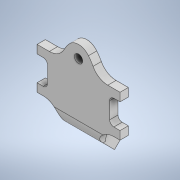
# Autodesk Inventor part: led_cap
Saved by Autodesk Inventor 2022 (Build 260153000, 153)
## iProperties
Created: 2024-07-06
Part Number: led_cap
Material: Типовые
Document SubType Name: Modeling
Designer: Капустяник Андрей
Density: 1 g/cm^3
Appearance: По умолчанию
Author: Капустяник Андрей
Autodesk Inventor part; units mm, degrees
ref_plane "YZ Plane" through (0, 0, 0) normal (1, 0, 0) x (0, 1, 0)
ref_plane "XZ Plane" through (0, 0, 0) normal (0, 1, 0) x (-1, 0, 0)
ref_plane "XY Plane" through (0, 0, 0) normal (0, 0, 1) x (1, 0, 0)
sketch "Эскиз1" plane through (0, 0, 0) normal (0, 0, 1) x (1, 0, 0)
  circle A0 centre (0, 0) radius 4.25
  line L0 (-4.5, 10) -> (4.5, 10)
  line L1 (4.5, 10) -> (4.5, -10)
  line L2 (4.5, -10) -> (-4.5, -10)
  line L3 (-4.5, -10) -> (-4.5, 10)
  line L4 (-4.5, 10) -> (4.5, -10) construction
  line L5 (4.5, 10) -> (-4.5, -10) construction
  dimension "d0" = 8.5
  dimension "d1" = 9
  dimension "d2" = 20
  constraints: 12 end point, 2 midpoint, 2 parallel, 1 centre point, 1 coincident, 1 horizontal, 1 perpendicular
  measures "d0" diameter of A0
  measures "d1" distance of L1.end L2.end
  measures "d2" distance of L0.end L1.end
extrude "Выдавливание1" add sketch "Эскиз1" along normal blind 2 contours A0 | L0 L1 L2 L3
sketch "Эскиз2" plane through (4.5, -10, 0) normal (1, 0, 0) x (0, 0, -1)
  line L0 (1.1161, 0) -> (2.1768, -1.0607) projected
  line L1 (3.9445, 0.7071) -> (2.1768, -1.0607) projected
  line L2 (3.9445, 0.7071) -> (2, 2.6517) projected
  line L3 (1.3283, 0.2121) -> (2.1768, -0.6364)
  line L4 (2.1768, -0.6364) -> (3.5203, 0.7071)
  line L5 (3.5203, 0.7071) -> (1.7879, 2.4395)
  line L6 (1.3283, 0.2121) -> (0, 1.5404)
  line L7 (0, 0) -> (0, 20) projected
  line L8 (1.7879, 2.4395) -> (0, 4.2274)
  point P0 (0, 10)
  dimension "d5" = 0.3
  constraints: 10 end point, 2 collinear, 2 point on line, 2 other
  measures "d5" distance between parallel lines of L1 L4
extrude "Выдавливание2" add sketch "Эскиз2" against normal up to surface (9 mm away)
sketch "Эскиз3" plane through (-4.5, -10, 2) normal (-1, 0, 0) x (0, 0, 1)
  line L0 (-2, 20) -> (-2, 4.2274) projected
  line L1 (-5.5203, 0.7071) -> (-2, 4.2274) projected
  line L2 (-4.1768, -0.6364) -> (-5.5203, 0.7071) projected
  line L3 (-2, 1.5404) -> (-4.1768, -0.6364) projected
  line L4 (-2, 1.5404) -> (-2, 0) projected
  line L5 (-2, 0) -> (0, 0) projected
  line L6 (0, 20) -> (0, 0) projected
  line L7 (-2, 20) -> (0, 20) projected
  line L8 (-2, 1.5404) -> (-2, 0) projected
  line L9 (-2, 1.5404) -> (0, 3.5404)
  line L10 (0, 20) -> (0, 0) projected
  point P0 (-2, 10)
  constraints: 3 point on line, 2 end point, 1 collinear
extrude "Выдавливание3" cut sketch "Эскиз3" against normal blind 10 contours L6 L5 L4 L9
sketch "Эскиз4" plane through (0, 0, 2) normal (0, 0, 1) x (1, 0, 0)
  arc A0 (4.03, 3.1777) -> (4.03, -0.8267) centre (0, 1.1755) ccw projected
  line L0 (0, 5.6755) -> (0, 10)
  line L1 (4.5, 10) -> (-4.5, 10) projected
  circle A1 centre (0, 8.1755) radius 1
  circle A2 centre (0, 8.1755) radius 2.5
  point P0 (0, 0)
  dimension "d10" = 2
  dimension "d14" = 5
  constraints: 2 centre point, 2 end point, 1 coincident, 1 midpoint, 1 point on circle, 1 point on line, 1 tangent
  measures "d10" diameter of A1
  measures "d14" diameter of A2
extrude "Выдавливание4" cut sketch "Эскиз4" against normal blind 10 contours A1 L0 | L0 A1
sketch "Эскиз5" plane through (0, 0, 2) normal (0, 0, 1) x (1, 0, 0)
  circle A0 centre (0, 8.1755) radius 1 projected
  circle A1 centre (0, 8.1755) radius 3
  point P0 (0, 0)
  dimension "d15" = 6
  constraints: 1 centre point, 1 coincident
  measures "d15" diameter of A1
extrude "Выдавливание5" add sketch "Эскиз5" against normal blind 2
fillet "Сопряжение1" radius 9 2 edges at (-4.5, 10, 1) (4.5, 10, 1)
fillet "Сопряжение2" radius 9 1 edges at (0, -5.7726, 0)
fillet "Сопряжение3" radius 4 1 edges at (0, -6.4596, 2)
sketch "Эскиз6" plane through (0, 0, 2) normal (0, 0, 1) x (1, 0, 0)
  circle A0 centre (0, 1.1755) radius 4 projected
  line L0 (-10, -3.8245) -> (10, -3.8245)
  line L1 (10, -3.8245) -> (10, 6.1755)
  line L2 (10, 6.1755) -> (-10, 6.1755)
  line L3 (-10, 6.1755) -> (-10, -3.8245)
  line L4 (-10, -3.8245) -> (10, 6.1755) construction
  line L5 (10, -3.8245) -> (-10, 6.1755) construction
  line L6 (7.5, 4.1755) -> (12.5, 4.1755)
  line L7 (12.5, 4.1755) -> (12.5, -1.8245)
  line L8 (12.5, -1.8245) -> (7.5, -1.8245)
  line L9 (7.5, -1.8245) -> (7.5, 4.1755)
  line L10 (7.5, 4.1755) -> (12.5, -1.8245) construction
  line L11 (12.5, 4.1755) -> (7.5, -1.8245) construction
  line L12 (-12.5, 4.1755) -> (-7.5, 4.1755)
  line L13 (-7.5, 4.1755) -> (-7.5, -1.8245)
  line L14 (-7.5, -1.8245) -> (-12.5, -1.8245)
  line L15 (-12.5, -1.8245) -> (-12.5, 4.1755)
  line L16 (-12.5, 4.1755) -> (-7.5, -1.8245) construction
  line L17 (-7.5, 4.1755) -> (-12.5, -1.8245) construction
  point P0 (0, 0)
  point P1 (10, 1.1755)
  point P2 (-10, 1.1755)
  point P3 (10, -1.8245)
  point P4 (10, 4.1755)
  point P5 (-10, 4.1755)
  point P6 (-10, -1.8245)
  dimension "d21" = 20
  dimension "d22" = 10
  dimension "d25" = 5
  dimension "d26" = 6
  dimension "d27" = 5
  dimension "d28" = 6
  constraints: 36 end point, 8 midpoint, 6 parallel, 3 horizontal, 3 perpendicular
  measures "d21" distance of L2.end L1.end
  measures "d22" distance of L1.end L0.end
  measures "d25" distance of L7.end L8.end
  measures "d26" distance of L6.end L7.end
  measures "d27" distance of L13.end L14.end
  measures "d28" distance of L12.end L13.end
extrude "Выдавливание6" add sketch "Эскиз6" against normal blind 2 contours A0 | L3 L14 L13 L12 L2 L1 L6 L9 L8 L0
fillet "Сопряжение4" radius 4 4 edges at (-4.2804, 6.1755, 1) (4.2804, 6.1755, 1) (-4.5, -3.8245, 1) (4.5, -3.8245, 1)
fillet "Сопряжение5" radius 1 4 edges at (-7.5, 4.1755, 1) (-7.5, -1.8245, 1) (7.5, 4.1755, 1) (7.5, -1.8245, 1)
